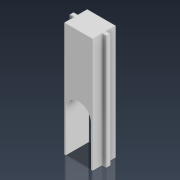
# Autodesk Inventor part: Slider-7
Saved by Autodesk Inventor 2021.1 (Build 251245010, 245A)
## iProperties
Created: 2020-12-20
Part Number: Slider-7
Material: 一般
Document SubType Name: Modeling
Designer: User
Density: 1 g/cm^3
Appearance: 預設
Author: User
Autodesk Inventor part; units mm, degrees
ref_plane "YZ Plane" through (0, 0, 0) normal (1, 0, 0) x (0, 1, 0)
ref_plane "XZ Plane" through (0, 0, 0) normal (0, 1, 0) x (-1, 0, 0)
ref_plane "XY Plane" through (0, 0, 0) normal (0, 0, 1) x (1, 0, 0)
sketch "草圖1" plane through (0, 0, 0) normal (0, 1, 0) x (-1, 0, 0)
  line L0 (-33.5, 27) -> (33.5, 27)
  line L1 (33.5, 27) -> (33.5, -27)
  line L2 (33.5, -27) -> (-33.5, -27)
  line L3 (-33.5, -27) -> (-33.5, 27)
  line L4 (-33.5, 27) -> (33.5, -27) construction
  line L5 (33.5, 27) -> (-33.5, -27) construction
  line L6 (43.5, -4.5) -> (33.5, -4.5)
  line L7 (33.5, -4.5) -> (33.5, 4.5)
  line L8 (33.5, 4.5) -> (43.5, 4.5)
  line L9 (43.5, 4.5) -> (43.5, -4.5)
  line L10 (-33.5, -4.5) -> (-43.5, -4.5)
  line L11 (-43.5, -4.5) -> (-43.5, 4.5)
  line L12 (-43.5, 4.5) -> (-33.5, 4.5)
  line L13 (-33.5, 4.5) -> (-33.5, -4.5)
  point P0 (0, 0)
  point P1 (33.5, 0)
  point P2 (-33.5, 0)
  point P3 (-33.5, 4.5)
  point P4 (-33.5, -4.5)
  dimension "d0" = 67
  dimension "d1" = 54
  dimension "d2" = 9
  dimension "d3" = 10
  constraints: 28 end point, 6 midpoint, 6 parallel, 3 horizontal, 3 perpendicular, 2 equal length
  measures "d0" distance of L0.start L0.end
  measures "d1" distance of L2.end L0.start
  measures "d2" distance of L8.end L6.start
  measures "d3" distance of L6.start L6.end
extrude "擠出1" add sketch "草圖1" along normal blind 400
sketch "草圖2" plane through (-33.5, 0, 27) normal (0, 0, 1) x (1, 0, 0)
  line L0 (0, 0) -> (0, 400) projected
  line L1 (0, 400) -> (67, 400) projected
  line L2 (67, 400) -> (67, 0) projected
  line L3 (67, 0) -> (0, 0) projected
  circle A0 centre (33.5, 199) radius 30
  line L4 (3.5, 199) -> (63.5, 199)
  line L5 (63.5, 199) -> (63.5, -2.327)
  line L6 (63.5, -2.327) -> (3.5, -2.327)
  line L7 (3.5, -2.327) -> (3.5, 199)
  point P0 (33.5, 0)
  point P1 (33.5, 0)
  point P2 (3.5, 199)
  point P3 (3.5, 0)
  point P4 (63.5, 0)
  dimension "d6" = 199
  dimension "d7" = 60
  constraints: 8 end point, 2 midpoint, 2 parallel, 1 centre point, 1 coincident, 1 horizontal, 1 perpendicular, 1 tangent, 1 vertical alignment
  measures "d6" distance from line of A0.centre L3
  measures "d7" diameter of A0
extrude "擠出2" cut sketch "草圖2" against normal through all contours L7 A0 L5 L3 | L4 A0 | A0 L4
sketch "草圖3" plane through (-33.5, 400, 27) normal (0, 0, 1) x (1, 0, 0)
  line L0 (-79.9627, -270) -> (146.9627, -270)
  line L1 (146.9627, -270) -> (146.9627, -400)
  line L2 (146.9627, -400) -> (-79.9627, -400)
  line L3 (-79.9627, -400) -> (-79.9627, -270)
  point P0 (33.5, -400)
  point P1 (33.5, -400)
  dimension "d10" = 130
  constraints: 8 end point, 2 parallel, 1 coincident, 1 horizontal, 1 midpoint, 1 perpendicular
  measures "d10" distance of L0.end L1.end
extrude "擠出3" cut sketch "草圖3" against normal through all
sketch "草圖4" plane through (33.5, 400, -27) normal (0, 0, -1) x (-1, 0, 0)
  arc A0 (63.5, -201) -> (3.5, -201) centre (33.5, -201) ccw construction
  circle A1 centre (33.5, -177) radius 30
  line L0 (63.5, -270) -> (3.5, -270)
  line L1 (3.5, -270) -> (3.5, -177)
  line L2 (3.5, -177) -> (63.5, -177)
  line L3 (63.5, -177) -> (63.5, -270)
  point P0 (33.5, -400)
  point P1 (63.5, -270)
  dimension "d13" = 24
  dimension "d14" = 60
  constraints: 8 end point, 2 coincident, 2 parallel, 1 centre point, 1 horizontal, 1 midpoint, 1 perpendicular, 1 tangent, 1 vertical alignment
  measures "d13" distance of A0.centre A1.centre
  measures "d14" diameter of A1
sketch "草圖5" plane through (-33.5, 400, 27) normal (0, 0, 1) x (1, 0, 0)
  circle A0 centre (33.5, -175) radius 30
  arc A1 (63.5, -201) -> (3.5, -201) centre (33.5, -201) ccw projected
  line L0 (63.5, -270) -> (3.5, -270)
  line L1 (3.5, -270) -> (3.5, -175)
  line L2 (3.5, -175) -> (63.5, -175)
  line L3 (63.5, -175) -> (63.5, -270)
  point P0 (33.5, -400)
  point P1 (63.5, -270)
  dimension "d15" = 26
  dimension "d16" = 60
  constraints: 8 end point, 2 coincident, 2 parallel, 1 centre point, 1 horizontal, 1 midpoint, 1 perpendicular, 1 tangent, 1 vertical alignment
  measures "d15" distance of A1.centre A0.centre
  measures "d16" diameter of A0
loft "斷面混成1" cut profiles "草圖4", "草圖5"
